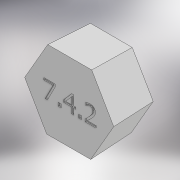
# Autodesk Inventor part: innerPosPlug1
Saved by Autodesk Inventor 2021 (Build 250183000, 183)
## iProperties
Created: 2020-07-05
Part Number: innerPosPlug1
Material: Generic
Document SubType Name: Modeling
Designer: Derm
Density: 1 g/cm^3
Appearance: Default
Author: Derm
Autodesk Inventor part; units mm, degrees
ref_plane "YZ Plane" through (0, 0, 0) normal (1, 0, 0) x (0, 1, 0)
ref_plane "XZ Plane" through (0, 0, 0) normal (0, 1, 0) x (-1, 0, 0)
ref_plane "XY Plane" through (0, 0, 0) normal (0, 0, 1) x (1, 0, 0)
sketch "Sketch1" plane through (0, 0, 0) normal (0, 0, 1) x (1, 0, 0)
  circle A0 centre (0, 0) radius 5.25 projected
  line L0 (4.7631, -8.25) -> (-4.7631, -8.25) projected
  line L1 (9.5263, 0) -> (4.7631, -8.25) projected
  line L2 (4.7631, 8.25) -> (9.5263, 0) projected
  line L3 (-4.7631, 8.25) -> (4.7631, 8.25) projected
  line L4 (-9.5263, 0) -> (-4.7631, 8.25) projected
  line L5 (-4.7631, -8.25) -> (-9.5263, 0) projected
  point P0 (0, 0)
extrude "Extrusion1" add sketch "Sketch1" along normal blind 9 contours A0 | L0 L5 L4 L3 L2 L1
draft "FaceDraft1" angle 2.5 pull direction (0, 0, -1) faces at (7.9386, 2.75, 3) (6.3509, -5.5, 3) (-1.5877, -8.25, 3) (-7.9386, -2.75, 3) (-6.3509, 5.5, 3) (1.5877, 8.25, 3) fixed edges at (7.1447, 4.125, 9) (7.1447, -4.125, 9) (0, -8.25, 0) (-7.1447, -4.125, 0) (-7.1447, 4.125, 9) (0, 8.25, 9)
shell "Shell1" thickness 1 removed faces 1 at (-3.1754, -0.262, 0)
sketch "Sketch3" plane through (0, 0, 9) normal (0, 0, 1) x (1, 0, 0)
  line L0 (-5.8305, -2.1571) -> (1.9852, -2.1571)
  line L1 (-3.1598, 1.0817) -> (-4.8086, -2.1571)
  line L2 (-4.8086, -2.1571) -> (-5.352, -2.1571)
  line L3 (-5.352, -2.1571) -> (-3.6106, 1.2052)
  line L4 (-3.6106, 1.2052) -> (-5.5773, 1.2052)
  line L5 (-5.5773, 1.2052) -> (-5.5773, 1.6529)
  line L6 (-5.5773, 1.6529) -> (-3.1598, 1.6529)
  line L7 (-3.1598, 1.6529) -> (-3.1598, 1.0817)
  line L8 (-1.8754, -2.1571) -> (-2.4867, -2.1571)
  line L9 (-2.4867, -2.1571) -> (-2.4867, -1.4285)
  line L10 (-2.4867, -1.4285) -> (-1.8754, -1.4285)
  line L11 (-1.8754, -1.4285) -> (-1.8754, -2.1571)
  line L12 (1.3449, -0.848) -> (0.891, -0.848)
  line L13 (0.891, -0.848) -> (0.891, -2.1571)
  line L14 (0.891, -2.1571) -> (0.4001, -2.1571)
  line L15 (0.4001, -2.1571) -> (0.4001, -0.848)
  line L16 (0.4001, -0.848) -> (-1.2826, -0.848)
  line L17 (-1.2826, -0.848) -> (-1.2826, -0.3108)
  line L18 (-1.2826, -0.3108) -> (0.4217, 1.6529)
  line L19 (0.4217, 1.6529) -> (0.891, 1.6529)
  line L20 (0.891, 1.6529) -> (0.891, -0.4374)
  line L21 (0.891, -0.4374) -> (1.3449, -0.4374)
  line L22 (1.3449, -0.4374) -> (1.3449, -0.848)
  line L23 (0.4001, -0.4374) -> (0.4001, 1.0508)
  line L24 (0.4001, 1.0508) -> (-0.8812, -0.4374)
  line L25 (-0.8812, -0.4374) -> (0.4001, -0.4374)
  line L26 (2.5706, -2.1571) -> (1.9593, -2.1571)
  line L27 (1.9593, -2.1571) -> (1.9593, -1.4285)
  line L28 (1.9593, -1.4285) -> (2.5706, -1.4285)
  line L29 (2.5706, -1.4285) -> (2.5706, -2.1571)
  line L30 (5.689, -2.1571) -> (3.3394, -2.1571)
  line L31 (3.3394, -2.1571) -> (3.3394, -1.6168)
  spline S0 degree 2 poles (3.3394, -1.6168) (3.5926, -1.3791) (4.0434, -0.9376) (4.2595, -0.6998) knots 0 0 0 1 2 2 2
  spline S1 degree 2 poles (4.2595, -0.6998) (4.6948, -0.2213) (5.0129, 0.353) (5.0129, 0.6587) knots 0 0 0 1 2 2 2
  spline S2 degree 2 poles (5.0129, 0.6587) (5.0129, 0.8192) (4.9141, 1.0601) (4.8245, 1.1372) knots 0 0 0 1 2 2 2
  spline S3 degree 2 poles (4.8245, 1.1372) (4.735, 1.2144) (4.5003, 1.2916) (4.3583, 1.2916) knots 0 0 0 1 2 2 2
  spline S4 degree 2 poles (4.3583, 1.2916) (4.2224, 1.2916) (3.9446, 1.2237) (3.818, 1.1712) knots 0 0 0 1 2 2 2
  spline S5 degree 2 poles (3.818, 1.1712) (3.7099, 1.128) (3.5092, 1.0045) (3.4475, 0.9613) knots 0 0 0 1 2 2 2
  line L32 (3.4475, 0.9613) -> (3.4197, 0.9613)
  line L33 (3.4197, 0.9613) -> (3.4197, 1.5047)
  spline S6 degree 2 poles (3.4197, 1.5047) (3.5772, 1.5819) (4.1422, 1.7331) (4.3953, 1.7331) knots 0 0 0 1 2 2 2
  spline S7 degree 2 poles (4.3953, 1.7331) (4.9295, 1.7331) (5.5316, 1.1681) (5.5316, 0.6865) knots 0 0 0 1 2 2 2
  spline S8 degree 2 poles (5.5316, 0.6865) (5.5316, 0.4611) (5.4266, 0.0844) (5.334, -0.0761) knots 0 0 0 1 2 2 2
  spline S9 degree 2 poles (5.334, -0.0761) (5.2413, -0.2429) (4.9727, -0.5702) (4.8245, -0.7276) knots 0 0 0 1 2 2 2
  spline S10 degree 2 poles (4.8245, -0.7276) (4.5837, -0.9901) (3.994, -1.552) (3.818, -1.7156) knots 0 0 0 1 2 2 2
  line L34 (3.818, -1.7156) -> (5.689, -1.7156)
  line L35 (5.689, -1.7156) -> (5.689, -2.1571)
  point P0 (0, 0)
  constraints: 2 end point, 2 horizontal
extrude "Extrusion2" cut sketch "Sketch3" against normal blind 0.2
body "Solid1"
